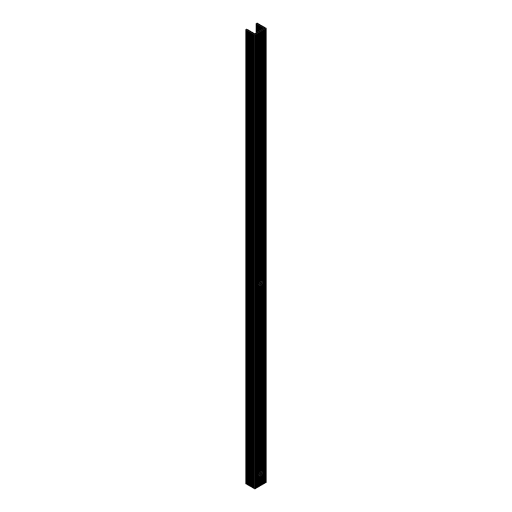
# Autodesk Inventor part: Stringer
Saved by Autodesk Inventor 2024 (Build 280153000, 153)
## iProperties
Created: 2023-12-30
Part Number: Stringer
Material: Aluminum
Document SubType Name: Modeling
Designer: Jamie
Density: 2.7 g/cm^3
Appearance: Satin
Author: Jamie
Autodesk Inventor part; units mm, degrees
ref_plane "YZ Plane" through (0, 0, 0) normal (1, 0, 0) x (0, 1, 0)
ref_plane "XZ Plane" through (0, 0, 0) normal (0, 1, 0) x (-1, 0, 0)
ref_plane "XY Plane" through (0, 0, 0) normal (0, 0, 1) x (1, 0, 0)
sketch "Sketch1" plane through (0, 0, 0) normal (0, 1, 0) x (-1, 0, 0)
  line L0 (0, 0) -> (8, 0)
  line L1 (8, -10) -> (0, -10)
  line L2 (0, -10) -> (0, 0)
  line L3 (8, -1) -> (1, -1)
  line L4 (1, -1) -> (1, -9)
  line L5 (1, -9) -> (8, -9)
  line L6 (8, 0) -> (8, -1)
  line L7 (8, -9) -> (8, -10)
  dimension "d0" = 1
  dimension "d1" = 1
  dimension "d2" = 1
  dimension "d3" = 10
  dimension "d4" = 8
  constraints: 16 end point, 4 parallel, 3 perpendicular, 2 horizontal, 1 collinear
  measures "d0" distance between parallel lines of L3 L0
  measures "d1" distance between parallel lines of L1 L5
  measures "d2" distance between parallel lines of L2 L4
  measures "d3" distance of L1.end L0.start
  measures "d4" distance of L0.start L0.end
extrude "Extrusion1" add sketch "Sketch1" along normal blind 339
sketch "Sketch2" plane through (0, 0, 0) normal (1, 0, 0) x (0, 0, -1)
  line L0 (0, 0) -> (10, 0) projected
  line L1 (0, 0) -> (0, 339) projected
  point P0 (5, 9)
  dimension "d7" = 9
  dimension "d8" = 5
  measures "d7" distance from line of L0 point (5, 9)
  measures "d8" distance from line of L1 point (5, 9)
hole "Hole1" at (0, 9, -5) direction (-1, 0, 0) diameter 3 depth 8 tip angle 118
sketch "Sketch3" plane through (0, 0, 0) normal (1, 0, 0) x (0, 0, -1)
  line L0 (0, 0) -> (0, 339) projected
  line L1 (0, 339) -> (10, 339) projected
  point P0 (5, 206.5)
  point P1 (5, 339)
  dimension "d16" = 5
  dimension "d17" = 132.5
  constraints: 1 midpoint
  measures "d16" distance from line of L0 point (5, 206.5)
  measures "d17" distance of point (5, 339) point (5, 206.5)
hole "Hole2" [suppressed]
sketch "Sketch5" plane through (0, 0, 0) normal (1, 0, 0) x (0, 0, -1)
  line L0 (0, 0) -> (0, 339) projected
  circle A0 centre (5, 9) radius 1.5 projected
  point P0 (5, 151)
  dimension "d25" = 5
  dimension "d26" = 142
  measures "d25" distance from line of L0 point (5, 151)
  measures "d26" distance of A0.centre point (5, 151)
hole "Hole3" at (0, 151, -5) direction (-1, 0, 0) diameter 3 depth 8 tip angle 118
body "Solid1"
